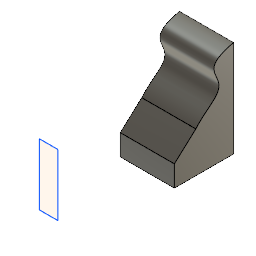
3.2 extrude extents (Autodesk Fusion 360 design; units mm, degrees)
Autodesk Fusion 360 part; units mm, degrees
sketch "Sketch2" plane through (0, 0, 0) normal (1, 0, 0) x (0, 1, 0)
  line L0 (0, 0) -> (0, 58.4328)
  line L1 (0, 58.4328) -> (35.9273, 58.4328)
  line L2 (35.9273, 58.4328) -> (35.9273, 45.6318)
  line L3 (35.9273, 45.6318) -> (22.9294, 33.8155)
  spline S0 degree 5 poles (22.9294, 33.8155) (22.6583, 33.4965) (22.1002, 32.8606) (21.2151, 31.9133) (19.9391, 30.663) (18.1926, 29.1199) (16.3243, 27.5908) (14.3973, 26.0642) (12.5198, 24.5199) (10.8609, 22.9268) (9.6061, 21.2511) (8.9082, 19.4651) (8.8442, 17.5557) (9.3551, 15.5351) (10.2337, 13.4436) (11.1928, 11.3365) (11.9149, 9.2744) (12.1049, 7.3137) (11.5522, 5.4947) (10.1339, 3.8407) (7.7859, 2.364) (5.1465, 1.3278) (2.7389, 0.6323) (0.9445, 0.2047) (0, 0) knots 0 0 0 0 0 0 0.05 0.1 0.15 0.2 0.25 0.3 0.35 0.4 0.45 0.5 0.55 0.6 0.65 0.7 0.75 0.8 0.85 0.9 0.95 1 1 1 1 1 1
extrude "Extrude1" add sketch "Sketch2" against normal blind 32.791
move_body "Move1" bodies 1 to x (1, 0, 0) y (0, -1, 0) z (0, 0, -1) at (0, 18.4141, 32.6691)
ref_plane "WorkPlane1" through (0, -76.691, 0) normal (0, 1, 0) x (0, 0, 1)
sketch "Sketch4" plane through (0, -76.691, 0) normal (0, 1, 0) x (1, 0, 0)
  line L0 (-22.4587, -18.5359) -> (-11.2332, -18.5359)
  line L1 (-11.2332, -18.5359) -> (-11.2332, 18.6854)
  line L2 (-11.2332, 18.6854) -> (-22.4587, 18.6854)
  line L3 (-22.4587, 18.6854) -> (-22.4587, -18.5359)
